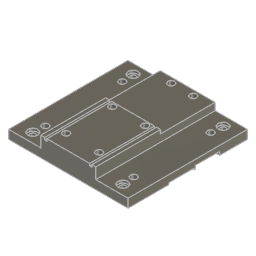
Assembly (Autodesk Fusion 360 archive; units mm, degrees)
design "Y_Stage_Prelim"
part number: 2026-04-23-15-36-49-562
Autodesk Fusion 360 part; units mm, degrees
note: some values were not read from the file. Chosen so that the rebuilt part matches the saved one: which face or edge a step refers to. Set by a fixed rule: which sketch regions a step uses.
sketch "Sketch1" plane through (0, 0, 0) normal (0, 0, 1) x (1, 0, 0)
  line L0 (-27.2, 27.2) -> (27.2, 27.2)
  line L1 (27.2, 27.2) -> (27.2, -27.2)
  line L2 (27.2, -27.2) -> (-27.2, -27.2)
  line L3 (-27.2, -27.2) -> (-27.2, 27.2)
  line L4 (-27.2, 27.2) -> (27.2, -27.2) construction
  line L5 (27.2, 27.2) -> (-27.2, -27.2) construction
  circle A0 centre (-20.1, 17.5) radius 1.5
  circle A1 centre (-20.1, -17.5) radius 1.5
  circle A2 centre (20.1, 17.5) radius 1.5
  circle A3 centre (20.1, -17.5) radius 1.5
  circle A4 centre (-4, 24.95) radius 1.5
  circle A5 centre (4, 24.95) radius 1.5
  circle A6 centre (-4, 7.95) radius 1.5
  circle A7 centre (4, 7.95) radius 1.5
  circle A8 centre (0, 10.7) radius 1.5
  dimension "d1" = 54.4
  dimension "d2" = 3
  dimension "d3" = 35
  dimension "d4" = 9.7
  dimension "d9" = 3
  dimension "d10" = 24.95
  dimension "d11" = 4
  dimension "d12" = 4
  dimension "d19" = 7.1
  dimension "d20" = 7.1
  dimension "d21" = 17
  dimension "d22" = 16.5
  dimension "d23" = 3
  constraint horizontal L0
  constraint perpendicular L0 L1
  constraint parallel L0 L2
  constraint parallel L1 L3
  constraint coincident L4 origin
  constraint coincident L5 origin
  constraint equal L0 L3
  constraint vertical A0.centre A1.centre
  constraint horizontal A1.centre A3.centre
  constraint vertical A2.centre A3.centre
  constraint horizontal A0.centre A2.centre
  constraint equal A0 A1
  constraint equal A1 A3
  constraint equal A2 A3
  constraint equal A4 A5
  constraint horizontal A4.centre A5.centre
  constraint vertical A5.centre A7.centre
  constraint vertical A4.centre A6.centre
  constraint equal A4 A6
  constraint equal A6 A7
  constraint horizontal A6.centre A7.centre
  constraint vertical origin A8.centre
  measures "d1" distance of L0.start L0.end
  measures "d2" diameter of A0
  measures "d3" distance of A0.centre A1.centre
  measures "d4" distance of L0 A0.centre
  measures "d9" diameter of A4
  measures "d10" vertical distance of origin A4.centre
  measures "d11" horizontal distance of origin A4.centre
  measures "d12" horizontal distance of origin A5.centre
  measures "d19" distance of L3 A0.centre
  measures "d20" distance of L1 A2.centre
  measures "d21" distance of A4.centre A6.centre
  measures "d22" distance of L0 A8.centre
  measures "d23" diameter of A8
extrude "Extrude1" add sketch "Sketch1" along normal blind 4 contours L0 L1 L2 L3 | A4 | A5 | A6 | A7 | A8
sketch "Sketch2" plane through (0, 0, 4) normal (0, 0, 1) x (-1, 0, 0)
  circle A0 centre (-20.1, 17.5) radius 1.5
  circle A1 centre (20.1, -17.5) radius 1.5
  circle A2 centre (20.1, 17.5) radius 1.5
  circle A3 centre (-20.1, -17.5) radius 1.5
  line L0 (27.2, 27.2) -> (-27.2, 27.2)
  line L1 (-27.2, 27.2) -> (-27.2, -27.2)
  line L2 (-27.2, -27.2) -> (27.2, -27.2)
  line L3 (27.2, -27.2) -> (27.2, 27.2)
  line L4 (12.5, -27.2) -> (-12.5, -27.2)
  line L5 (-12.5, -27.2) -> (-12.5, 27.2)
  line L6 (-12.5, 27.2) -> (12.5, 27.2)
  line L7 (12.5, 27.2) -> (12.5, -27.2)
  line L8 (12.5, -27.2) -> (-12.5, 27.2) construction
  line L9 (-12.5, -27.2) -> (12.5, 27.2) construction
  dimension "d13" = 25
  constraint horizontal L4
  constraint perpendicular L4 L5
  constraint parallel L4 L6
  constraint parallel L5 L7
  constraint coincident L8 origin
  constraint coincident L9 origin
  constraint coincident L2 L4.start
  measures "d13" distance of L4.start L4.end
extrude "Extrude2" add sketch "Sketch2" along normal blind 3 contours L0 L2 L4 L5 L6 L7
sketch "Sketch5" plane through (0, 0, 7) normal (0, 0, 1) x (-1, 0, 0)
  line L0 (12.5, 27.2) -> (-12.5, 27.2)
  line L1 (-12.5, 27.2) -> (-12.5, -27.2)
  line L2 (-12.5, -27.2) -> (12.5, -27.2)
  line L3 (12.5, -27.2) -> (12.5, 27.2)
  circle A0 centre (7.5, -0.3) radius 1.5
  circle A1 centre (-7.5, -0.3) radius 1.5
  circle A2 centre (7.5, 20.7) radius 1.5
  circle A3 centre (-7.5, 20.7) radius 1.5
  circle A4 centre (5, -24.7) radius 1.5
  circle A5 centre (-5, -24.7) radius 1.5
  circle A6 centre (5, -10.7) radius 1.5
  circle A7 centre (-5, -10.7) radius 1.5
  dimension "d27" = 15
  dimension "d28" = 21
  dimension "d29" = 3
  dimension "d31" = 7.5
  dimension "d34" = 10
  dimension "d35" = 14
  dimension "d36" = 3
  dimension "d37" = 5
  dimension "d38" = 2.5
  dimension "d49" = 26.9
  constraint vertical A0.centre A2.centre
  constraint horizontal A0.centre A1.centre
  constraint horizontal A2.centre A3.centre
  constraint vertical A1.centre A3.centre
  constraint equal A2 A3
  constraint equal A0 A2
  constraint equal A0 A1
  constraint vertical A4.centre A6.centre
  constraint horizontal A6.centre A7.centre
  constraint vertical A5.centre A7.centre
  constraint horizontal A4.centre A5.centre
  constraint equal A4 A5
  constraint equal A5 A7
  constraint equal A6 A7
  measures "d27" distance of A0.centre A1.centre
  measures "d28" distance of A0.centre A2.centre
  measures "d29" diameter of A0
  measures "d31" horizontal distance of origin A2.centre
  measures "d34" distance of A4.centre A5.centre
  measures "d35" vertical distance of A4.centre A6.centre
  measures "d36" diameter of A4
  measures "d37" horizontal distance of origin A4.centre
  measures "d38" distance of L2 A4.centre
  measures "d49" distance of L2 A0.centre
extrude "Extrude5" cut sketch "Sketch5" against normal blind 3 contours A0 | A1 | A2 | A3 | A4 | A5
sketch "Sketch6" plane through (0, 0, 7) normal (0, 0, 1) x (-1, 0, 0)
  line L0 (12.5, 27.2) -> (-12.5, 27.2)
  line L1 (-12.5, 27.2) -> (-12.5, -27.2)
  line L2 (-12.5, -27.2) -> (12.5, -27.2)
  line L3 (12.5, -27.2) -> (12.5, 27.2)
  circle A0 centre (5, -24.7) radius 1.5
  circle A1 centre (7.5, 20.7) radius 1.5
  circle A2 centre (7.5, -0.3) radius 1.5
  circle A3 centre (-5, -24.7) radius 1.5
  circle A4 centre (-7.5, 20.7) radius 1.5
  circle A5 centre (-7.5, -0.3) radius 1.5
  line L4 (12.5, 27.2) -> (-12.5, 27.2)
  line L5 (-12.5, 27.2) -> (-12.5, -2.3)
  line L6 (-12.5, -2.3) -> (12.5, -2.3)
  line L7 (12.5, -2.3) -> (12.5, 27.2)
  dimension "d39" = 29.5
  constraint horizontal L4
  constraint vertical L5
  constraint horizontal L6
  constraint vertical L7
  constraint coincident L1 L5.end
  constraint coincident L0.start L3.end
  measures "d39" distance of L0.start L6.end
extrude "Extrude6" add sketch "Sketch6" along normal blind 2 contours L0 L1 L3 L4 L5 L6 L7
extrude "Extrude8" add 1 faces at (1.484, 9.3012, 7) along direction (0, 0, 1) blind 0.3
sketch "Sketch8" plane through (0, 0, 9) normal (0, 0, 1) x (-1, 0, 0)
  circle A0 centre (7.5, -0.3) radius 1.5
  circle A1 centre (7.5, 20.7) radius 1.5
  circle A2 centre (-7.5, 20.7) radius 1.5
  circle A3 centre (-7.5, -0.3) radius 1.5
  line L0 (12.5, -2.3) -> (12.5, 27.2)
  line L1 (12.5, 27.2) -> (-12.5, 27.2)
  line L2 (-12.5, 27.2) -> (-12.5, -2.3)
  line L3 (-12.5, -2.3) -> (12.5, -2.3)
  line L4 (10.73, -2.3) -> (9.73, -2.3)
  line L5 (9.73, -2.3) -> (9.73, 27.2)
  line L6 (9.73, 27.2) -> (10.73, 27.2)
  line L7 (10.73, 27.2) -> (10.73, -2.3)
  line L8 (-9.73, -2.3) -> (-10.73, -2.3)
  line L9 (-10.73, -2.3) -> (-10.73, 27.2)
  line L10 (-10.73, 27.2) -> (-9.73, 27.2)
  line L11 (-9.73, 27.2) -> (-9.73, -2.3)
  dimension "d52" = 1
  dimension "d53" = 1.77
  dimension "d54" = 1.77
  constraint horizontal L4
  constraint vertical L5
  constraint horizontal L6
  constraint vertical L7
  constraint coincident L1 L5.end
  constraint coincident L3 L4.start
  constraint horizontal L8
  constraint vertical L9
  constraint horizontal L10
  constraint vertical L11
  constraint coincident L1 L9.end
  constraint coincident L3 L8.start
  constraint equal L4 L8
  measures "d52" distance of L4.start L4.end
  measures "d53" distance of L0 L7
  measures "d54" distance of L2 L9
extrude "Extrude9" cut sketch "Sketch8" against normal blind 1 contours L1 L3 L4 L5 L6 L7 | L1 L3 L8 L9 L10 L11
sketch "Sketch9" plane through (0, 0, 0) normal (0, 0, -1) x (1, 0, 0)
  circle A0 centre (20.1, 17.5) radius 1.5
  circle A1 centre (-20.1, 17.5) radius 1.5
  circle A2 centre (20.1, -17.5) radius 1.5
  circle A3 centre (-20.1, -17.5) radius 1.5
  line L0 (27.2, 27.2) -> (-27.2, 27.2)
  line L1 (-27.2, 27.2) -> (-27.2, -27.2)
  line L2 (-27.2, -27.2) -> (27.2, -27.2)
  line L3 (27.2, -27.2) -> (27.2, 27.2)
  circle A4 centre (-20.5, 22.85) radius 1.25
  circle A5 centre (20.5, 22.85) radius 1.25
  circle A6 centre (-20.5, -22.85) radius 1.25
  circle A7 centre (20.5, -22.85) radius 1.25
  dimension "d57" = 41
  dimension "d58" = 45.7
  dimension "d59" = 2.5
  dimension "d60" = 20.5
  dimension "d61" = 22.85
  constraint equal A6 A7
  constraint equal A4 A6
  constraint equal A4 A5
  constraint horizontal A4.centre A5.centre
  constraint vertical A5.centre A7.centre
  constraint horizontal A6.centre A7.centre
  constraint vertical A4.centre A6.centre
  measures "d57" distance of A4.centre A5.centre
  measures "d58" distance of A4.centre A6.centre
  measures "d59" diameter of A6
  measures "d60" horizontal distance of origin A6.centre
  measures "d61" vertical distance of origin A4.centre
extrude "Extrude10" cut sketch "Sketch9" against normal blind 5 contours A4 | A5 | A6 | A7
sketch "Sketch10" plane through (0, 0, 4) normal (0, 0, 1) x (-1, 0, 0)
  circle A0 centre (20.5, 22.85) radius 1.25
  circle A1 centre (20.5, -22.85) radius 1.25
  line L0 (12.5, 27.2) -> (12.5, -27.2)
  line L1 (12.5, -27.2) -> (27.2, -27.2)
  line L2 (27.2, -27.2) -> (27.2, 27.2)
  line L3 (27.2, 27.2) -> (12.5, 27.2)
  circle A2 centre (20.1, 17.5) radius 1.5
  circle A3 centre (20.1, -17.5) radius 1.5
  circle A4 centre (20.5, -22.85) radius 2.25
  circle A5 centre (20.5, 22.85) radius 2.25
  circle A6 centre (-20.5, 22.85) radius 2.25
  circle A7 centre (-20.5, 22.85) radius 1.25
  circle A8 centre (-20.5, -22.85) radius 2.25
  circle A9 centre (-20.5, -22.85) radius 1.25
  dimension "d64" = 4.5
  constraint concentric A1 A4
  constraint concentric A0 A5
  constraint concentric A6 A7
  constraint concentric A8 A9
  constraint equal A5 A6
  constraint equal A4 A6
  constraint equal A4 A8
  measures "d64" diameter of A8
extrude "Extrude11" cut sketch "Sketch10" against normal blind 1.15 contours A4 | A5 | A6 | A8
sketch "Sketch11" plane through (0, 0, 0) normal (0, 0, -1) x (1, 0, 0)
  line L0 (27.2, 27.2) -> (-27.2, 27.2)
  line L1 (-27.2, 27.2) -> (-27.2, -27.2)
  line L2 (-27.2, -27.2) -> (27.2, -27.2)
  line L3 (27.2, -27.2) -> (27.2, 27.2)
  circle A0 centre (-20.1, -17.5) radius 1.5
  circle A1 centre (20.1, -17.5) radius 1.5
  circle A2 centre (-20.1, 17.5) radius 1.5
  circle A3 centre (20.1, 17.5) radius 1.5
  circle A4 centre (20.5, -22.85) radius 1.25
  circle A5 centre (-20.5, -22.85) radius 1.25
  circle A6 centre (20.5, 22.85) radius 1.25
  circle A7 centre (-20.5, 22.85) radius 1.25
  line L4 (-27.2, -14.5) -> (27.2, -14.5)
  line L5 (27.2, -14.5) -> (27.2, -3.5)
  line L6 (27.2, -3.5) -> (-27.2, -3.5)
  line L7 (-27.2, -3.5) -> (-27.2, -14.5)
  dimension "d67" = 11
  dimension "d68" = 12.7
  constraint horizontal L4
  constraint vertical L5
  constraint horizontal L6
  constraint vertical L7
  constraint coincident L3 L5.end
  constraint coincident L1 L4.start
  measures "d67" distance of L4.start L6.end
  measures "d68" distance of L2 L4
extrude "Extrude12" cut sketch "Sketch11" against normal blind 1.6 contours L1 L3 L4 L5 L6 L7
sketch "Sketch12" plane through (0, 0, 0) normal (0, 0, -1) x (1, 0, 0)
  line L0 (-27.2, -3.5) -> (27.2, -3.5)
  line L1 (27.2, -3.5) -> (27.2, 27.2)
  line L2 (27.2, 27.2) -> (-27.2, 27.2)
  line L3 (-27.2, 27.2) -> (-27.2, -3.5)
  circle A0 centre (-20.5, 22.85) radius 1.25
  circle A1 centre (20.5, 22.85) radius 1.25
  circle A2 centre (20.1, 17.5) radius 1.5
  circle A3 centre (-20.1, 17.5) radius 1.5
  line L4 (27.2, -3) -> (-27.2, -3)
  line L5 (-27.2, -3) -> (-27.2, 8.5)
  line L6 (-27.2, 8.5) -> (27.2, 8.5)
  line L7 (27.2, 8.5) -> (27.2, -3)
  line L8 (-27.2, -27.2) -> (27.2, -27.2)
  dimension "d71" = 11.5
  dimension "d72" = 24.2
  constraint horizontal L4
  constraint vertical L5
  constraint horizontal L6
  constraint vertical L7
  constraint coincident L3 L5.end
  constraint coincident L1 L4.start
  measures "d71" distance of L4.start L6.end
  measures "d72" distance of L4 L8
extrude "Extrude13" cut sketch "Sketch12" against normal blind 0.8 contours L1 L3 L4 L5 L6 L7
ref_plane "WorkPlane1" through (0, 0, 1.5) normal (-1, 0, 0) x (0, -1, 0)
sketch "Sketch7" plane through (0, 0, 0) normal (-1, 0, 0) x (0, -1, 0)
  line L0 (27.2, 0) -> (27.2, 8.1)
  line L1 (27.2, 8.1) -> (17.2, 8.1)
  line L2 (17.2, 8.1) -> (9.1, 0)
  line L3 (9.1, 0) -> (27.2, 0)
  line L4 (-2.3, 8.1) -> (27.2, 8.1)
  line L5 (27.2, 3) -> (12.1, 3)
  line L6 (12.1, 3) -> (12.1, 0)
  point P0 (27.2, 8.1)
  point P1 (27.2, 0)
  dimension "d42" = 10
  dimension "d43" = 45
  dimension "d46" = 3
  constraint vertical L0
  constraint perpendicular L0 L1
  constraint horizontal L3
  constraint coincident P0 L0.end
  constraint coincident L0.start L3.end
  constraint coincident L0 L5.start
  constraint coincident L2 L5.end
  constraint perpendicular L0 L5
  constraint coincident L3 L6.end
  constraint perpendicular L3 L6
  measures "d42" distance of P0 L1.end
  measures "d43" angle of L2 L4
  measures "d46" distance of L3 L5
extrude "Extrude7" [suppressed]
sketch "Sketch4" plane through (0, 0, 0) normal (0, 0, -1) x (1, 0, 0)
  circle A0 centre (20.4, 17.5) radius 1.5
  circle A1 centre (0, -11) radius 1.5
  circle A2 centre (-5, -9.3) radius 1.5
  circle A3 centre (5, -9.3) radius 1.5
  circle A4 centre (-20.4, -17.5) radius 1.5
  circle A5 centre (20.4, -17.5) radius 1.5
  circle A6 centre (-5, -25) radius 1.5
  circle A7 centre (5, -25) radius 1.5
  line L0 (27.5, 27.5) -> (-27.5, 27.5)
  line L1 (-27.5, 27.5) -> (-27.5, -27.5)
  line L2 (-27.5, -27.5) -> (27.5, -27.5)
  line L3 (27.5, -27.5) -> (27.5, 27.5)
  circle A8 centre (-20.4, 17.5) radius 1.5
  circle A9 centre (0, -11) radius 2.5
  dimension "d24" = 5
  constraint concentric A1 A9
  measures "d24" diameter of A9
extrude "Extrude4" [suppressed]
sketch "Sketch3" plane through (0, 0, 6) normal (0, 0, 1) x (-1, 0, 0)
  circle A0 centre (-5, -20) radius 1.5
  circle A1 centre (5, -20) radius 1.5
  line L0 (10.3, 25) -> (-10.3, 25)
  line L1 (-10.3, 25) -> (-10.3, -25)
  line L2 (-10.3, -25) -> (10.3, -25)
  line L3 (10.3, -25) -> (10.3, 25)
  line L4 (10.3, 25) -> (-10.3, 25)
  line L5 (-10.3, 25) -> (-10.3, 20)
  line L6 (-10.3, 20) -> (10.3, 20)
  line L7 (10.3, 20) -> (10.3, 25)
  dimension "d16" = 5
  constraint horizontal L4
  constraint vertical L5
  constraint horizontal L6
  constraint vertical L7
  constraint coincident L1 L5.end
  constraint coincident L0.start L3.end
  measures "d16" distance of L0.end L5.end
extrude "Extrude3" [suppressed]
equation "d4 = ( d1 - d3 ) / 2"
equation "d5 = 26 mm + 1.9 mm - 2.5 mm"
equation "d10 = 25 mm - 0.95 mm + 1.2 mm - 0.3 mm"
equation "d12 = d11"
equation "d19 = d20"
equation "d22 = 14 mm + 2.5 mm"
equation "d23 = d9"
equation "d31 = d27 / 2"
equation "d37 = d34 / 2"
equation "d60 = d57 / 2"
equation "d61 = d58 / 2"

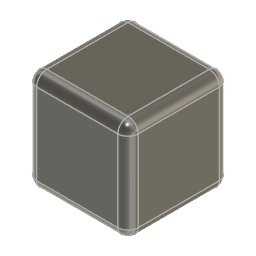
design "Magnet"
part number: 2026-04-23-09-43-52-141
Autodesk Fusion 360 part; units mm, degrees
sketch "Sketch1" plane through (0, 0, 0) normal (0, 0, 1) x (1, 0, 0)
  line L0 (18.5072, 2.4976) -> (23.5072, 2.4976)
  line L1 (23.5072, 2.4976) -> (23.5072, -2.5024)
  line L2 (23.5072, -2.5024) -> (18.5072, -2.5024)
  line L3 (18.5072, -2.5024) -> (18.5072, 2.4976)
  line L4 (18.5072, 2.4976) -> (23.5072, -2.5024) construction
  line L5 (23.5072, 2.4976) -> (18.5072, -2.5024) construction
  point P0 (21.0072, -0.0024)
  dimension "d3" = 5
  dimension "d4" = 5
  constraint horizontal L0
  constraint perpendicular L0 L1
  constraint parallel L0 L2
  constraint parallel L1 L3
  constraint coincident L4 P0
  constraint coincident L5 P0
  measures "d3" distance of L0.start L2.end
  measures "d4" distance of L0.start L0.end
extrude "Extrude1" add sketch "Sketch1" along normal blind 5
fillet "Fillet1" radius 0.5 12 edges at (23.5072, -0.0024, 5) (21.0072, -2.5024, 5) (23.5072, -2.5024, 2.5) (23.5072, -0.0024, 0) (21.0072, -2.5024, 0) (18.5072, -2.5024, 2.5) (18.5072, -0.0024, 5) (18.5072, -0.0024, 0) (18.5072, 2.4976, 2.5) (21.0072, 2.4976, 5) (23.5072, 2.4976, 2.5) (21.0072, 2.4976, 0)
equation "d4 = d3"

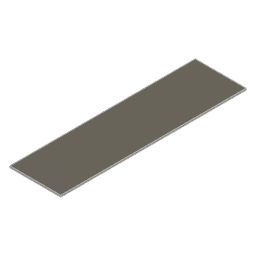
design "EI_Magnet_Shim"
part number: 2026-05-03-19-46-17-008
Autodesk Fusion 360 part; units mm, degrees
sketch "Sketch1" plane through (0, 0, 0) normal (0, 0, 1) x (1, 0, 0)
  line L0 (0, 40) -> (11, 40)
  line L1 (11, 40) -> (11, 0)
  line L2 (11, 0) -> (0, 0)
  line L3 (0, 0) -> (0, 40)
  dimension "d1" = 11
  dimension "d2" = 40
  constraint horizontal L0
  constraint perpendicular L0 L1
  constraint parallel L0 L2
  constraint parallel L1 L3
  constraint coincident L2.end L3.start
  measures "d1" distance of L0.start L0.end
  measures "d2" distance of L0.end L1.end
extrude "Extrude1" add sketch "Sketch1" along normal blind 0.35

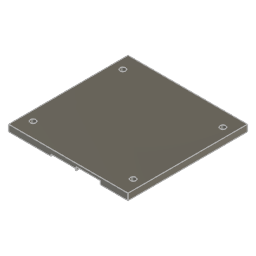
design "Sample_Stage_Prelim"
part number: 2026-04-23-15-36-49-562
Autodesk Fusion 360 part; units mm, degrees
sketch "Sketch1" plane through (0, 0, 0) normal (0, 0, 1) x (1, 0, 0)
  line L0 (-27.3, 27.3) -> (27.3, 27.3)
  line L1 (27.3, 27.3) -> (27.3, -27.3)
  line L2 (27.3, -27.3) -> (-27.3, -27.3)
  line L3 (-27.3, -27.3) -> (-27.3, 27.3)
  line L4 (-27.3, 27.3) -> (27.3, -27.3) construction
  line L5 (27.3, 27.3) -> (-27.3, -27.3) construction
  circle A0 centre (-22.85, 20.5) radius 1.25
  circle A1 centre (-22.85, -20.5) radius 1.25
  circle A2 centre (22.85, 20.5) radius 1.25
  circle A3 centre (22.85, -20.5) radius 1.25
  circle A4 centre (-5, 20) radius 1.25
  circle A5 centre (5, 20) radius 1.25
  circle A6 centre (-17.35, 20.5) radius 1.25
  circle A7 centre (-17.35, -20.5) radius 1.25
  circle A8 centre (17.35, -20.5) radius 1.25
  circle A9 centre (17.35, 20.5) radius 1.25
  dimension "d1" = 54.6
  dimension "d2" = 2.5
  dimension "d3" = 41
  dimension "d9" = 2.5
  dimension "d10" = 20
  dimension "d11" = 5
  dimension "d12" = 5
  dimension "d16" = 5.5
  dimension "d17" = 5.5
  dimension "d34" = 45.7
  dimension "d42" = 22.85
  dimension "d43" = 20.5
  constraint horizontal L0
  constraint perpendicular L0 L1
  constraint parallel L0 L2
  constraint parallel L1 L3
  constraint coincident L4 origin
  constraint coincident L5 origin
  constraint equal L0 L3
  constraint vertical A0.centre A1.centre
  constraint horizontal A1.centre A3.centre
  constraint vertical A2.centre A3.centre
  constraint horizontal A0.centre A2.centre
  constraint equal A0 A1
  constraint equal A1 A3
  constraint equal A2 A3
  constraint equal A4 A5
  constraint horizontal A4.centre A5.centre
  constraint equal A6 A9
  constraint equal A2 A9
  constraint equal A2 A8
  constraint equal A7 A8
  constraint horizontal A0.centre A6.centre
  constraint vertical A6.centre A7.centre
  constraint horizontal A1.centre A7.centre
  constraint horizontal A7.centre A8.centre
  constraint vertical A8.centre A9.centre
  constraint horizontal A2.centre A9.centre
  measures "d1" distance of L0.start L0.end
  measures "d2" diameter of A0
  measures "d3" distance of A0.centre A1.centre
  measures "d9" diameter of A4
  measures "d10" vertical distance of origin A4.centre
  measures "d11" horizontal distance of origin A4.centre
  measures "d12" horizontal distance of origin A5.centre
  measures "d16" distance of A0.centre A6.centre
  measures "d17" distance of A2.centre A9.centre
  measures "d34" distance of A0.centre A2.centre
  measures "d42" horizontal distance of origin A0.centre
  measures "d43" vertical distance of origin A0.centre
extrude "Extrude1" add sketch "Sketch1" along normal blind 3 contours L0 L1 L2 L3 | A4 | A5 | A6 | A7 | A8 | A9
sketch "Sketch9" plane through (0, -27.3, 0) normal (0, -1, 0) x (1, 0, 0)
  line L0 (-27.3, 0) -> (27.3, 0)
  line L1 (27.3, 0) -> (27.3, 3)
  line L2 (27.3, 3) -> (-27.3, 3)
  line L3 (-27.3, 3) -> (-27.3, 0)
  line L4 (-3.1, 0) -> (-3.25, 0.3)
  line L5 (-3.25, 0.3) -> (3.25, 0.3)
  line L6 (3.25, 0.3) -> (3.1, 0)
  dimension "d44" = 0.15
  dimension "d45" = 0.3
  dimension "d46" = 6.5
  dimension "d56" = 3.25
  constraint coincident L0 L4.start
  constraint parallel L0 L5
  constraint coincident L0 L6.end
  constraint equal L4 L6
  measures "d44" horizontal distance of L5.end L6.end
  measures "d45" vertical distance of L5.end L6.end
  measures "d46" distance of L4.end L5.end
  measures "d56" horizontal distance of origin L4.end
extrude "Extrude7" cut sketch "Sketch9" against normal blind 55 contours L0 L4 L5 L6
sketch "Sketch10" plane through (0, 0, 0) normal (0, 0, -1) x (1, 0, 0)
  line L0 (-3.1, -27.3) -> (-3.1, 27.3)
  line L1 (-3.1, 27.3) -> (-27.3, 27.3)
  line L2 (-27.3, 27.3) -> (-27.3, -27.3)
  line L3 (-27.3, -27.3) -> (-3.1, -27.3)
  line L4 (27.3, -27.3) -> (27.3, 27.3)
  line L5 (27.3, 27.3) -> (3.1, 27.3)
  line L6 (3.1, 27.3) -> (3.1, -27.3)
  circle A0 centre (-22.85, 20.5) radius 1.25
  circle A1 centre (-22.85, -20.5) radius 1.25
  circle A2 centre (22.85, -20.5) radius 1.25
  circle A3 centre (22.85, 20.5) radius 1.25
  line L7 (14.6, -27.3) -> (3.6, -27.3)
  line L8 (3.6, -27.3) -> (3.6, 27.7)
  line L9 (3.6, 27.7) -> (14.6, 27.7)
  line L10 (14.6, 27.7) -> (14.6, -27.3)
  line L11 (3.1, -27.3) -> (27.3, -27.3)
  dimension "d50" = 11
  dimension "d51" = 55
  dimension "d53" = 0.5
  constraint horizontal L7
  constraint vertical L8
  constraint horizontal L9
  constraint vertical L10
  constraint coincident L3 L7.start
  measures "d50" distance of L8.end L9.end
  measures "d51" distance of L7.start L9.end
  measures "d53" distance of L6 L8
extrude "Extrude8" cut sketch "Sketch10" against normal blind 1.6 contours L5 L7 L8 L10 L11 | L5 L8 L9 L10
sketch "Sketch11" plane through (0, 0, 0) normal (0, 0, -1) x (1, 0, 0)
  line L0 (27.3, 27.3) -> (14.6, 27.3)
  line L1 (-3.1, -27.3) -> (-3.1, 27.3)
  line L2 (-3.1, 27.3) -> (-27.3, 27.3)
  line L3 (-27.3, 27.3) -> (-27.3, -27.3)
  line L4 (-27.3, -27.3) -> (-3.1, -27.3)
  circle A0 centre (-22.85, 20.5) radius 1.25
  circle A1 centre (-22.85, -20.5) radius 1.25
  line L5 (3.1, -27.3) -> (-7.9, -27.3)
  line L6 (-7.9, -27.3) -> (-7.9, 27.3)
  line L7 (-7.9, 27.3) -> (3.1, 27.3)
  line L8 (3.1, 27.3) -> (3.1, -27.3)
  line L9 (14.6, 27.3) -> (14.6, -27.3)
  line L10 (14.6, -27.3) -> (27.3, -27.3)
  line L11 (27.3, -27.3) -> (27.3, 27.3)
  circle A2 centre (22.85, -20.5) radius 1.25
  circle A3 centre (22.85, 20.5) radius 1.25
  line L12 (3.25, -27.3) -> (-3.25, -27.3)
  dimension "d57" = 4.8
  constraint horizontal L5
  constraint vertical L6
  constraint horizontal L7
  constraint vertical L8
  constraint coincident L2 L6.end
  constraint collinear L5 L12
  measures "d57" distance of L1 L6
extrude "Extrude9" cut sketch "Sketch11" against normal blind 0.8 contours L1 L2 L4 L5 L6 L7 L12 | L1 L5 L7 L8 L12
sketch "Sketch5" plane through (0, 0, 0) normal (0, 0, -1) x (1, 0, 0)
  line L0 (25, 25) -> (-25, 25)
  line L1 (-25, 25) -> (-25, -25)
  line L2 (-25, -25) -> (25, -25)
  line L3 (25, -25) -> (25, 25)
  circle A0 centre (-15.15, -20.5) radius 1.25
  circle A1 centre (20.65, 20.5) radius 1.25
  circle A2 centre (-20.65, -20.5) radius 1.25
  circle A3 centre (-15.15, 20.5) radius 1.25
  circle A4 centre (20.65, -20.5) radius 1.25
  circle A5 centre (15.15, -20.5) radius 1.25
  circle A6 centre (15.15, 20.5) radius 1.25
  circle A7 centre (-20.65, 20.5) radius 1.25
  line L4 (25, -25) -> (-25, -25)
  line L5 (-25, -25) -> (-25, 25)
  line L6 (-25, 25) -> (25, 25)
  line L7 (25, 25) -> (25, -25)
  constraint horizontal L4
  constraint vertical L5
  constraint horizontal L6
  constraint vertical L7
  constraint coincident L0.end L1.start
  constraint coincident L2.end L3.start
sketch "Sketch6" plane through (0, 0, 3) normal (0, 0, 1) x (-1, 0, 0)
  line L0 (27.5, 27.5) -> (-27.5, 27.5)
  line L1 (-27.5, 27.5) -> (-27.5, -27.5)
  line L2 (-27.5, -27.5) -> (27.5, -27.5)
  line L3 (27.5, -27.5) -> (27.5, 27.5)
  circle A0 centre (23.15, 20.5) radius 1.25
  circle A1 centre (23.15, -20.5) radius 1.25
  line L4 (-27.5, -12.8) -> (27.5, -12.8)
  line L5 (27.5, -12.8) -> (27.5, 12.8)
  line L6 (27.5, 12.8) -> (-27.5, 12.8)
  line L7 (-27.5, 12.8) -> (-27.5, -12.8)
  line L8 (-27.5, -12.8) -> (27.5, 12.8) construction
  line L9 (27.5, -12.8) -> (-27.5, 12.8) construction
  circle A2 centre (-23.15, 20.5) radius 1.25
  circle A3 centre (-23.15, -20.5) radius 1.25
  dimension "d23" = 25.6
  constraint horizontal L4
  constraint perpendicular L4 L5
  constraint parallel L4 L6
  constraint parallel L5 L7
  constraint coincident L8 origin
  constraint coincident L9 origin
  constraint coincident L1 L4.start
  measures "d23" distance of L4.start L6.end
extrude "Extrude4" [suppressed]
sketch "Sketch7" plane through (0, 0, 0) normal (0, 0, -1) x (1, 0, 0)
  line L0 (27.5, 27.5) -> (-27.5, 27.5)
  line L1 (-27.5, 27.5) -> (-27.5, -27.5)
  line L2 (-27.5, -27.5) -> (27.5, -27.5)
  line L3 (27.5, -27.5) -> (27.5, 27.5)
  circle A0 centre (-23.15, 20.5) radius 1.25
  circle A1 centre (-23.15, -20.5) radius 1.25
  circle A2 centre (17.5, -20.4) radius 1.5
  circle A3 centre (-17.5, -20.4) radius 1.5
  circle A4 centre (17.5, 20.4) radius 1.5
  circle A5 centre (-17.5, 20.4) radius 1.5
  circle A6 centre (23.15, 20.5) radius 1.25
  circle A7 centre (23.15, -20.5) radius 1.25
  dimension "d26" = 35
  dimension "d27" = 40.8
  dimension "d28" = 3
  dimension "d29" = 20.4
  dimension "d30" = 17.5
  constraint equal A4 A5
  constraint equal A2 A4
  constraint equal A2 A3
  constraint vertical A2.centre A4.centre
  constraint horizontal A4.centre A5.centre
  constraint vertical A3.centre A5.centre
  constraint horizontal A2.centre A3.centre
  measures "d26" distance of A2.centre A3.centre
  measures "d27" distance of A2.centre A4.centre
  measures "d28" diameter of A4
  measures "d29" vertical distance of origin A4.centre
  measures "d30" horizontal distance of origin A2.centre
extrude "Extrude5" [suppressed]
sketch "Sketch8" plane through (0, 0, 6) normal (0, 0, 1) x (-1, 0, 0)
  line L0 (-27.5, 12.8) -> (-27.5, -12.8)
  line L1 (-27.5, -12.8) -> (27.5, -12.8)
  line L2 (27.5, -12.8) -> (27.5, 12.8)
  line L3 (27.5, 12.8) -> (-27.5, 12.8)
  circle A0 centre (25, -5) radius 1.5
  circle A1 centre (25, 5) radius 1.5
  circle A2 centre (9.3, 5) radius 1.5
  circle A3 centre (9.3, -5) radius 1.5
  dimension "d35" = 15.7
  dimension "d36" = 10
  dimension "d37" = 3
  dimension "d38" = 5
  dimension "d39" = 2.5
  constraint vertical A0.centre A1.centre
  constraint horizontal A1.centre A2.centre
  constraint vertical A2.centre A3.centre
  constraint horizontal A0.centre A3.centre
  constraint equal A2 A3
  constraint equal A1 A2
  constraint equal A0 A1
  measures "d35" horizontal distance of A0.centre A3.centre
  measures "d36" vertical distance of A0.centre A1.centre
  measures "d37" diameter of A0
  measures "d38" vertical distance of origin A3.centre
  measures "d39" distance of L2 A0.centre
extrude "Extrude6" [suppressed]
equation "d2 = d9"
equation "d5 = 20 mm - 2.1 mm"
equation "d12 = d11"
equation "d17 = d16"
equation "d29 = d27 / 2"
equation "d30 = d26 / 2"
equation "d38 = d36 / 2"
equation "d42 = d34 / 2"
equation "d43 = d3 / 2"
equation "d56 = d46 / 2"
equation "d57 = 11 mm - 6.2 mm"

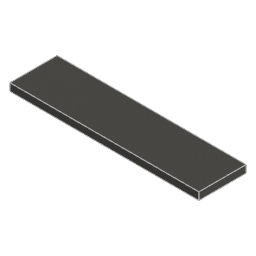
design "Magnetic Tape"
part number: 2025-07-22-16-52-46-665
Autodesk Fusion 360 part; units mm, degrees
sketch "Sketch1" plane through (0, 0, 0) normal (0, 0, 1) x (1, 0, 0)
  line L0 (-20, 5) -> (20, 5)
  line L1 (20, 5) -> (20, -5)
  line L2 (20, -5) -> (-20, -5)
  line L3 (-20, -5) -> (-20, 5)
  line L4 (-20, 5) -> (20, -5) construction
  line L5 (20, 5) -> (-20, -5) construction
  dimension "d1" = 10
  dimension "d2" = 40
  constraint horizontal L0
  constraint perpendicular L0 L1
  constraint parallel L0 L2
  constraint parallel L1 L3
  constraint coincident L4 origin
  constraint coincident L5 origin
  measures "d1" distance of L0.start L2.end
  measures "d2" distance of L0.start L0.end
extrude "Extrude1" add sketch "Sketch1" along normal blind 1.6

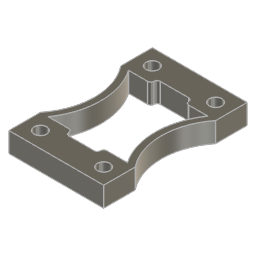
design "Flexure Mount"
part number: 2026-04-23-12-48-19-527
Autodesk Fusion 360 part; units mm, degrees
sketch "Sketch1" plane through (0, 0, 0) normal (0, 0, 1) x (1, 0, 0)
  line L0 (-7.5, 6.35) -> (7.5, 6.35)
  line L1 (7.5, 6.35) -> (7.5, 11.35)
  line L2 (7.5, 11.35) -> (-7.5, 11.35)
  line L3 (-7.5, 11.35) -> (-7.5, 6.35)
  line L4 (-7.5, 6.35) -> (7.5, 11.35) construction
  line L5 (7.5, 6.35) -> (-7.5, 11.35) construction
  line L6 (-7.5, -6.35) -> (7.5, -6.35)
  line L7 (7.5, -6.35) -> (7.5, -11.35)
  line L8 (7.5, -11.35) -> (-7.5, -11.35)
  line L9 (-7.5, -11.35) -> (-7.5, -6.35)
  line L10 (-7.5, -6.35) -> (7.5, -11.35) construction
  line L11 (7.5, -6.35) -> (-7.5, -11.35) construction
  arc A0 (-7.5, -6.35) -> (-7.5, 6.35) centre (-15.5, 0) ccw
  arc A1 (-6.2573, -6.35) -> (-6.2573, 6.35) centre (-15.5, 0) ccw
  arc A2 (7.5, 6.35) -> (7.5, -6.35) centre (15.5, 0) ccw
  arc A3 (6.2573, 6.35) -> (6.2573, -6.35) centre (15.5, 0) ccw
  circle A4 centre (-5, -8.85) radius 1
  circle A5 centre (5, -8.85) radius 1
  line L12 (-2.75, 6.35) -> (2.75, 6.35)
  line L13 (2.75, 6.35) -> (2.75, 7.35)
  line L14 (2.75, 7.35) -> (-2.75, 7.35)
  line L15 (-2.75, 7.35) -> (-2.75, 6.35)
  line L16 (-2.75, 6.35) -> (2.75, 7.35) construction
  line L17 (2.75, 6.35) -> (-2.75, 7.35) construction
  line L18 (-2.5, -6.35) -> (2.5, -6.35)
  line L19 (2.5, -6.35) -> (2.5, -7.35)
  line L20 (2.5, -7.35) -> (-2.5, -7.35)
  line L21 (-2.5, -7.35) -> (-2.5, -6.35)
  line L22 (-2.5, -6.35) -> (2.5, -7.35) construction
  line L23 (2.5, -6.35) -> (-2.5, -7.35) construction
  line L24 (0, 0) -> (-9.3045, 0) construction
  circle A6 centre (-5, 8.85) radius 1
  circle A7 centre (5, 8.85) radius 1
  point P0 (0, 8.85)
  point P1 (0, -8.85)
  point P2 (0, 6.85)
  point P3 (0, -6.85)
  dimension "d3" = 15
  dimension "d4" = 5
  dimension "d5" = 6.35
  dimension "d6" = 6.35
  dimension "d8" = 1
  dimension "d13" = 1
  dimension "d14" = 8
  dimension "d15" = 8
  dimension "d16" = 2
  dimension "d17" = 5
  dimension "d18" = 5
  dimension "d19" = 5.5
  dimension "d20" = 1
  dimension "d21" = 1
  dimension "d22" = 5
  constraint horizontal L0
  constraint perpendicular L0 L1
  constraint parallel L0 L2
  constraint parallel L1 L3
  constraint coincident L4 P0
  constraint coincident L5 P0
  constraint horizontal L6
  constraint perpendicular L6 L7
  constraint parallel L6 L8
  constraint parallel L7 L9
  constraint coincident L10 P1
  constraint coincident L11 P1
  constraint equal L0 L6
  constraint equal L3 L9
  constraint vertical L24.start P0
  constraint vertical L24.start P1
  constraint coincident L6 A1.start
  constraint coincident A0.centre A1.centre
  constraint coincident L6 A3.end
  constraint coincident L0 A3.start
  constraint coincident A2.centre A3.centre
  constraint horizontal L24.start A2.centre
  constraint coincident L6.end L7.start
  constraint coincident L0 A1.end
  constraint equal A4 A5
  constraint horizontal P1 A4.centre
  constraint horizontal P1 A5.centre
  constraint horizontal L12
  constraint perpendicular L12 L13
  constraint parallel L12 L14
  constraint parallel L13 L15
  constraint coincident L16 P2
  constraint coincident L17 P2
  constraint coincident L0 L12.start
  constraint horizontal L18
  constraint perpendicular L18 L19
  constraint parallel L18 L20
  constraint parallel L19 L21
  constraint coincident L22 P3
  constraint coincident L23 P3
  constraint coincident L6 L18.start
  constraint vertical L24.start P2
  constraint vertical L24.start P3
  constraint coincident L24.start origin
  constraint horizontal L24
  constraint symmetric A4 L24 A6
  constraint symmetric A5 L24 A7
  measures "d3" distance of L1.end L2.end
  measures "d4" distance of L0.start L2.end
  measures "d5" distance of L24.start L6
  measures "d6" distance of L24.start L0
  measures "d8" distance of A2 A3
  measures "d13" distance of A0 A1
  measures "d14" horizontal distance of L0.start A0.centre
  measures "d15" horizontal distance of L0.end A2.centre
  measures "d16" diameter of A5
  measures "d17" distance of P1 A4.centre
  measures "d18" distance of P1 A5.centre
  measures "d19" distance of L13.end L14.end
  measures "d20" distance of L12.end L13.end
  measures "d21" distance of L18.end L19.end
  measures "d22" distance of L19.end L20.end
extrude "Extrude1" add sketch "Sketch1" along normal blind 3.175 contours L0 L1 L2 L3 L13 L14 L15 | L0 L6 A0 A1 | L6 L7 L8 L9 L19 L20 L21 | L0 L6 A2 A3
fillet "Fillet1" radius 0.5 8 edges at (-2.5, -7.35, 1.5875) (-2.5, -6.35, 1.5875) (-2.75, 6.35, 1.5875) (-2.75, 7.35, 1.5875) (2.75, 6.35, 1.5875) (2.75, 7.35, 1.5875) (2.5, -6.35, 1.5875) (2.5, -7.35, 1.5875)
sketch "Sketch3" plane through (0, 0, 3.175) normal (0, 0, 1) x (-1, 0, 0)
  circle A0 centre (-5, -8.85) radius 1
  circle A1 centre (5, -8.85) radius 1
  circle A2 centre (5, 8.85) radius 1
  arc A3 (-3, 6.35) -> (-2.5, 6.85) centre (-3, 6.85) ccw
  arc A4 (-2, 7.35) -> (-2.5, 6.85) centre (-2, 6.85) ccw
  line L0 (-2, 7.35) -> (2, 7.35)
  arc A5 (2.5, 6.85) -> (2, 7.35) centre (2, 6.85) ccw
  arc A6 (2.5, 6.85) -> (3, 6.35) centre (3, 6.85) ccw
  line L1 (3, 6.35) -> (6.2573, 6.35)
  arc A7 (6.2573, 6.35) -> (6.2573, -6.35) centre (15.5, 0) ccw
  line L2 (6.2573, -6.35) -> (3.25, -6.35)
  arc A8 (3.25, -6.35) -> (2.75, -6.85) centre (3.25, -6.85) ccw
  arc A9 (2.25, -7.35) -> (2.75, -6.85) centre (2.25, -6.85) ccw
  line L3 (2.25, -7.35) -> (-2.25, -7.35)
  arc A10 (-2.75, -6.85) -> (-2.25, -7.35) centre (-2.25, -6.85) ccw
  arc A11 (-2.75, -6.85) -> (-3.25, -6.35) centre (-3.25, -6.85) ccw
  line L4 (-3.25, -6.35) -> (-6.2573, -6.35)
  arc A12 (-6.2573, -6.35) -> (-6.2573, 6.35) centre (-15.5, 0) ccw
  line L5 (-6.2573, 6.35) -> (-3, 6.35)
  circle A13 centre (-5, 8.85) radius 1
  line L6 (-7.5, -11.35) -> (7.5, -11.35)
  line L7 (7.5, -11.35) -> (7.5, -6.35)
  arc A14 (7.5, 6.35) -> (7.5, -6.35) centre (15.5, 0) ccw
  line L8 (7.5, 6.35) -> (7.5, 11.35)
  line L9 (7.5, 11.35) -> (-7.5, 11.35)
  line L10 (-7.5, 11.35) -> (-7.5, 6.35)
  arc A15 (-7.5, -6.35) -> (-7.5, 6.35) centre (-15.5, 0) ccw
  line L11 (-7.5, -6.35) -> (-7.5, -11.35)
  circle A16 centre (5, 8.85) radius 1
  constraint concentric A2 A16
equation "d6 = d5"
equation "d8 = d13"
equation "d11 = 0'- 1/8\""
equation "d15 = d14"
equation "d18 = d17"
equation "d21 = d20"
